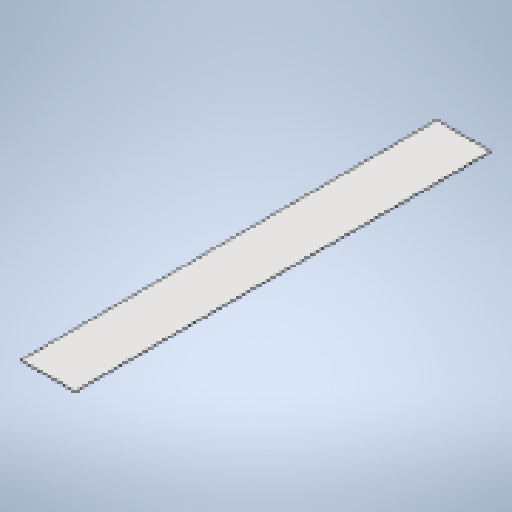
# Autodesk Inventor part: GnG frame 1.1 floor sheet 5
Saved by Autodesk Inventor 2025.3 (Build 293356030, 356C)
## iProperties
Created: 2025-10-28
Part Number: GnG frame 1.1 floor sheet 5
Material: Stainless Steel
Document SubType Name: Sheet Metal
Designer: admin
Mass: 280.619 g
Surface Area: 364.406 cm^2
Volume: 35.0774 cm^3
Density: 8 g/cm^3
Sheet Metal Rule: AISI304 3mm Die 32
Sheet Metal Width: 300,000 mm
Sheet Metal Length: 2300,000 mm
Sheet Metal Area: 690000,000 mm^2
Appearance: Default
Stock Number: 1.5
Flat Pattern Width: 30 cm
Flat Pattern Length: 230 cm
Flat Pattern Area: 6900 cm^2
Author: admin
Autodesk Inventor part; units mm, degrees
ref_plane "YZ Plane" through (0, 0, 0) normal (1, 0, 0) x (0, 1, 0)
ref_plane "XZ Plane" through (0, 0, 0) normal (0, 1, 0) x (-1, 0, 0)
ref_plane "XY Plane" through (0, 0, 0) normal (0, 0, 1) x (1, 0, 0)
sketch "Sketch1" plane through (0, 0, 0) normal (0, 0, 1) x (1, 0, 0)
  line L0 (0, 0) -> (-300, 0)
  line L1 (-300, 0) -> (-300, -2300)
  line L2 (-300, -2300) -> (0, -2300)
  line L3 (0, -2300) -> (0, 0)
  line L4 (0, 0) -> (-40, 0)
  line L5 (-40, 0) -> (-40, -40)
  line L6 (-40, -40) -> (0, -40)
  line L7 (0, -40) -> (0, 0)
  line L8 (0, -2300) -> (-40, -2300)
  line L9 (-40, -2300) -> (-40, -2260)
  line L10 (-40, -2260) -> (0, -2260)
  line L11 (0, -2260) -> (0, -2300)
  line L12 (-300, 0) -> (-260, 0)
  line L13 (-260, 0) -> (-260, -40)
  line L14 (-260, -40) -> (-300, -40)
  line L15 (-300, -40) -> (-300, 0)
  line L16 (-300, -2300) -> (-260, -2300)
  line L17 (-260, -2300) -> (-260, -2260)
  line L18 (-260, -2260) -> (-300, -2260)
  line L19 (-300, -2260) -> (-300, -2300)
  line L20 (-220, -2300) -> (-130, -2300)
  line L21 (-130, -2300) -> (-130, -2260)
  line L22 (-130, -2260) -> (-220, -2260)
  line L23 (-220, -2260) -> (-220, -2300)
  line L24 (-220, 0) -> (-130, 0)
  line L25 (-130, 0) -> (-130, -40)
  line L26 (-130, -40) -> (-220, -40)
  line L27 (-220, -40) -> (-220, 0)
  point P0 (0, -40)
  point P1 (-40, 0)
  point P2 (-40, -2300)
  point P3 (0, -2260)
  point P4 (-130, 0)
  point P5 (-260, 0)
  point P6 (-300, -40)
  dimension "d22" = 300
  dimension "d23" = 2300
  dimension "d24" = 40
  dimension "d25" = 40
  dimension "d28" = 90
  dimension "d29" = 90
  measures "d22" distance of L2.end L1.end
  measures "d23" distance of L1.end L0.end
  measures "d24" distance of L6.end L5.end
  measures "d25" distance of L5.end L4.end
  measures "d28" distance of L25.end L26.end
  measures "d29" distance between parallel lines of L5 L25
extrude "Plate1" add sketch "Sketch1" along normal blind 3
sketch "Sketch5" plane through (0, 0, 3) normal (0, 0, 1) x (1, 0, 0)
  line L0 (0, 0) -> (-100, 0) construction
  line L1 (-100, 0) -> (-100, -5) construction
  line L2 (-100, -5) -> (0, -5) construction
  line L3 (0, -5) -> (0, 0) construction
  line L4 (-100, 0) -> (-101.3084, -4.1277)
  arc A0 (-103.6916, -4.1277) -> (-101.3084, -4.1277) centre (-102.5, -3.75) ccw
  line L5 (-103.6916, -4.1277) -> (-105, 0)
  line L6 (-105, 0) -> (-100, 0)
  line L7 (-105, 0) -> (-110, 0) construction
  line L8 (-110, 0) -> (-115, 0)
  line L9 (-115, 0) -> (-115, -5)
  line L10 (-115, -5) -> (-110, -5)
  line L11 (-110, -5) -> (-110, 0)
  line L12 (-115, 0) -> (-120, 0) construction
  line L13 (-120, 0) -> (-125, 0)
  line L14 (-125, 0) -> (-125, -5)
  line L15 (-125, -5) -> (-120, -5)
  line L16 (-120, -5) -> (-120, 0)
  line L17 (-125, 0) -> (-130, 0) construction
  line L18 (-130, 0) -> (-135, 0)
  line L19 (-135, 0) -> (-135, -5)
  line L20 (-135, -5) -> (-130, -5)
  line L21 (-130, -5) -> (-130, 0)
  line L22 (-135, 0) -> (-140, 0) construction
  line L23 (-140, 0) -> (-145, 0)
  line L24 (-145, 0) -> (-145, -5)
  line L25 (-145, -5) -> (-140, -5)
  line L26 (-140, -5) -> (-140, 0)
  line L27 (-145, 0) -> (-150, 0) construction
  line L28 (-150, 0) -> (-155, 0) construction
  circle A1 centre (-150, 0) radius 2.5
  point P0 (-102.5, 0)
  dimension "d31" = 100
  dimension "d32" = 5
  dimension "d33" = 5
  dimension "d34" = 5
  dimension "d35" = 1.25
  dimension "d36" = 5
  dimension "d37" = 5
  dimension "d38" = 5
  dimension "d39" = 5
  constraints: 58 end point, 11 horizontal, 10 equal length, 10 parallel, 5 perpendicular, 3 tangent, 2 centre point, 2 coincident, 2 point on circle, 1 midpoint, 1 point on line, 1 vertical alignment
  measures "d31" distance of L2.end L1.end
  measures "d32" distance of L1.end L0.end
  measures "d33" distance of L9.end L8.end
  measures "d34" distance of L5.end L0.end
  measures "d35" radius of A0
  measures "d36" distance of L14.end L13.end
  measures "d37" distance of L19.end L18.end
  measures "d38" distance of L24.end L23.end
  measures "d39" diameter of A1
extrude "Cut1" cut sketch "Sketch5" against normal blind 3 contours L4 A0 L5 L6 | A1
equation "\"d35\" = 0.25 * d32"
equation "\"d39\" = d32"
equation "\"d40\" = Thickness"
equation "\"d2\" = Thickness"
equation "\"BendReliefWidth\" = Thickness"
equation "\"BendReliefDepth\" = 0.5 * Thickness"
equation "\"CornerReliefSize\" = 4 * Thickness"
equation "\"MinimumRemnant\" = 2 * Thickness"
equation "\"TransitionRadius\" = BendRadius"
equation "\"JacobiRadiusSize\" = BendRadius"
equation "\"GapSize\" = Thickness"
equation "\"Thickness\" = 3"
equation "\"BendRadius\" = 5"
body "Solid1"
